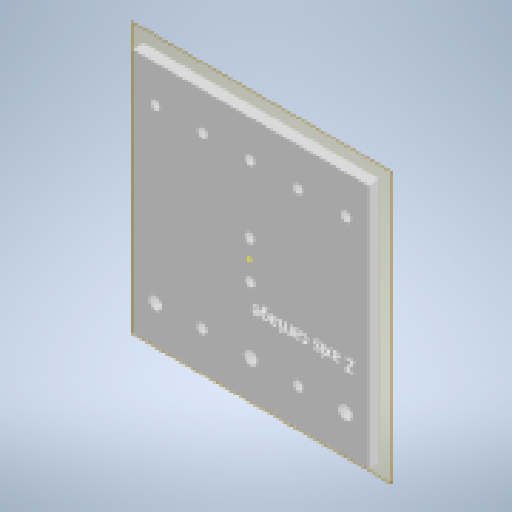
# Autodesk Inventor part: X axis carriage small 2
Saved by Autodesk Inventor 2023.2 (Build 272271000, 271)
## iProperties
Created: 2023-05-10
Part Number: X axis carriage small 2
Material: Generic
Document SubType Name: Modeling
Designer: dmargari
Density: 1 g/cm^3
Appearance: Default
Author: dmargari
Autodesk Inventor part; units mm, degrees
ref_plane "YZ Plane" through (0, 0, 0) normal (1, 0, 0) x (0, 1, 0)
ref_plane "XZ Plane" through (0, 0, 0) normal (0, 1, 0) x (-1, 0, 0)
ref_plane "XY Plane" through (0, 0, 0) normal (0, 0, 1) x (1, 0, 0)
ref_plane "Work Plane1" through (0, 0, 0) normal (0, 0, 1) x (1, 0, 0)
sketch "Sketch1" plane through (0, 0, 0) normal (0, 0, 1) x (1, 0, 0)
  line L0 (-62.5, -65) -> (-62.5, 65) projected
  line L1 (62.5, -65) -> (-62.5, -65) projected
  line L2 (-62.5, 65) -> (62.5, 65) projected
  line L3 (62.5, 65) -> (62.5, -65) projected
  circle A0 centre (50.2, 45) radius 2.55 projected
  circle A1 centre (50.2, -45) radius 3.55 projected
  circle A2 centre (-50.2, -45) radius 2.55 projected
  circle A3 centre (-50.2, 45) radius 2.55 projected
  line L4 (-50.2, -87.1872) -> (-50.2, 86.9163) construction
  line L5 (0, -90.5792) -> (0, 86.9163) construction
  line L6 (50.2, -82.9351) -> (50.2, 98.888) construction
  line L7 (-25.1, -100.0293) -> (-25.1, 98.888) construction
  line L8 (25.1, -87.1872) -> (25.1, 98.888) construction
  line L9 (-84.1215, -10) -> (86.0151, -10) construction
  line L10 (-84.1215, 10) -> (86.0151, 10) construction
  point P0 (0, 0)
  point P1 (0, 45)
  point P2 (0, -45)
  point P3 (-25.1, -45)
  point P4 (25.1, -45)
  point P5 (25.1, 45)
  point P6 (-25.1, 45)
  point P7 (0, 0)
  point P8 (0, -10)
  point P9 (0, 10)
  dimension "d0" = 100.4
  dimension "d1" = 50.2
  dimension "d2" = 25.1
  dimension "d3" = 25.1
  dimension "d4" = 10
  dimension "d5" = 20
  constraints: 14 end point, 10 point on line, 5 coincident, 5 vertical, 1 parallel, 1 perpendicular
  measures "d0" distance between parallel lines of L4 L6
  measures "d1" distance between parallel lines of L4 L5
  measures "d2" distance between parallel lines of L5 L7
  measures "d3" distance between parallel lines of L5 L8
  measures "d4" distance from line of point (0, 0) L9
  measures "d5" distance between parallel lines of L9 L10
extrude "Extrusion1" add sketch "Sketch1" along normal blind 6 contours L0 L2 L3 L1 | A0 | A1 | A2 | A3
sketch "Sketch2" plane through (0, 0, 0) normal (0, 0, -1) x (-1, 0, 0)
  point P0 (0, 0)
  point P1 (-50.176, -44.9419)
  point P2 (-0.1594, -45.1078)
  point P3 (50.2816, -45.0688)
hole "Hole1" at (50.176, -44.9419, 0) at (0.1594, -45.1078, 0) at (-50.2816, -45.0688, 0) direction (0, 0, 1) diameter 7.1 end through all counterbore diameter 7.5 counterbore depth 2
sketch "Sketch3" plane through (0, 0, 0) normal (0, 0, -1) x (-1, 0, 0)
  point P0 (0, 0)
  point P1 (50.3086, 45.5821)
  point P2 (0.2433, 45.4506)
  point P3 (-50.5722, 44.8972)
hole "Hole2" at (-50.3086, 45.5821, 0) at (-0.2433, 45.4506, 0) at (50.5722, 44.8972, 0) direction (0, 0, 1) diameter 5.1 end through all counterbore diameter 7.5 counterbore depth 2
sketch "Sketch4" plane through (0, 0, 0) normal (0, 0, -1) x (-1, 0, 0)
  point P0 (0, 0)
  point P1 (25.3396, 45.2378)
  point P2 (-25.1139, 44.8345)
  point P3 (-25.1745, -45.3838)
  point P4 (25.6326, -44.5055)
  point P5 (0.0949, -10.3157)
  point P6 (0.3775, 9.6536)
hole "Hole3" at (25.1139, 44.8345, 0) at (-25.3396, 45.2378, 0) at (25.1745, -45.3838, 0) at (-25.6326, -44.5055, 0) at (-0.0949, -10.3157, 0) at (-0.3775, 9.6536, 0) direction (0, 0, 1) diameter 5.1 end through all
sketch "Sketch5" plane through (0, 0, 6) normal (0, 0, 1) x (1, 0, 0)
  line L0 (54.8683, -25.7428) -> (1.0212, -25.7428) construction
  line L1 (1.0212, -25.7428) -> (1.0212, -17.8731) construction
  line L2 (1.0212, -17.8731) -> (54.8683, -17.8731) construction
  line L3 (54.8683, -17.8731) -> (54.8683, -25.7428) construction
  point P0 (0, 0)
  constraints: 2 other
equation "\"d1\" = 0.5 * d0"
equation "\"d2\" = 0.5 * d1"
equation "\"d3\" = d2"
body "Solid1"
